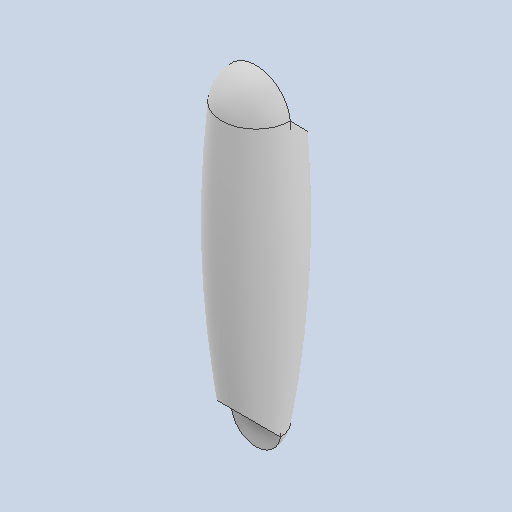
# Autodesk Inventor part: ч ASY human dummy 01
Saved by Autodesk Inventor 2024.2 (Build 282272000, 272)
## iProperties
Created: 2020-06-29
Part Number: ч ASY human dummy 01
Material: Типовые
Document SubType Name: Modeling
Designer: admin
Density: 1 g/cm^3
Appearance: По умолчанию
Author: admin
Autodesk Inventor part; units mm, degrees
ref_plane "YZ Plane" through (0, 0, 0) normal (1, 0, 0) x (0, 1, 0)
ref_plane "XZ Plane" through (0, 0, 0) normal (0, 1, 0) x (-1, 0, 0)
ref_plane "XY Plane" through (0, 0, 0) normal (0, 0, 1) x (1, 0, 0)
sketch "Эскиз1" plane through (0, 0, 0) normal (0, 0, 1) x (1, 0, 0)
  arc A0 (0, -52) -> (51.771881, 4.865426) centre (0, 0) ccw construction
  arc A1 (0, -447.5) -> (36.997666, -416.117411) centre (0, -410) ccw
  arc A2 (36.997666, -416.117411) -> (51.771881, 4.865426) centre (-1581.033587, -148.582622) ccw
  line L0 (0, 126.427921) -> (0, -660.016615)
  arc A3 (0, 52) -> (0, -52) centre (0, 0) ccw construction
  arc A4 (0, -372.5) -> (0, -447.5) centre (0, -410) ccw construction
  arc A5 (51.771881, 4.865426) -> (0, 52) centre (0, 0) ccw
  arc A6 (36.997666, -416.117411) -> (0, -372.5) centre (0, -410) ccw construction
  point P0 (0, -266.794347)
  dimension "d0" = 104
  dimension "d1" = 75
  dimension "d2" = 410
  dimension "d3" = 1640
  constraints: 14 point on circle, 7 centre point, 4 point on line, 2 end point, 2 tangent, 2 vertical alignment, 1 coincident, 1 midpoint, 1 vertical
  measures "d0" diameter of A0
  measures "d1" diameter of A1
  measures "d2" distance of A1.centre point (0, 0)
  measures "d3" radius of A2
revolve "Вращение1" add sketch "Эскиз1" angle 360 about axis through (0, 126.427921, 0) along (0, -1, 0)
sketch "Эскиз2" plane through (0, 0, 0) normal (0, 0, 1) x (1, 0, 0)
  circle A0 centre (0, 0) radius 52
  dimension "d5" = 104
  constraints: 1 centre point, 1 coincident
  measures "d5" diameter of A0
extrude "Выдавливание1" cut sketch "Эскиз2" against normal through all
sketch "Эскиз3" plane through (0, 0, 0) normal (0, 0, 1) x (1, 0, 0)
  circle A0 centre (0, -410) radius 37.5
  point P0 (0, 0)
  dimension "d8" = 410
  dimension "d9" = 75
  constraints: 1 centre point, 1 vertical alignment
  measures "d8" distance of point (0, 0) A0.centre
  measures "d9" diameter of A0
extrude "Выдавливание2" cut sketch "Эскиз3" along normal through all
equation "\"d0\" = knee_diam"
equation "\"d1\" = feet_joint_diam"
equation "\"d2\" = surae"
equation "\"d3\" = 4 * surae"
equation "\"d5\" = knee_diam"
equation "\"d8\" = surae"
equation "\"d9\" = feet_joint_diam"
equation "\"knee_diam\" = 104"
equation "\"feet_joint_diam\" = 75"
equation "\"surae\" = 410"
